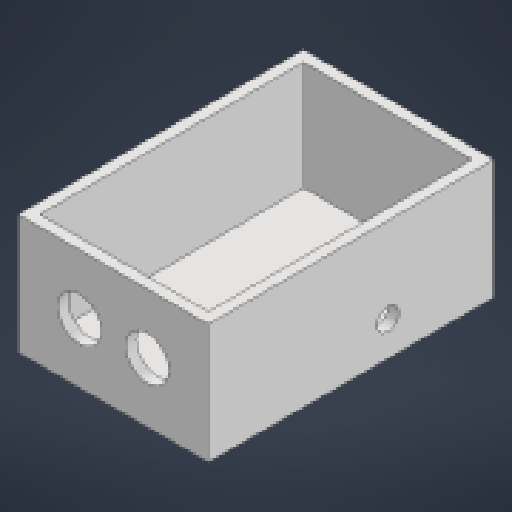
# Autodesk Inventor part: Prototipo
Saved by Autodesk Inventor 2026 (Build 300175050, 175E)
## iProperties
Created: 2025-09-06
Part Number: Prototipo
Material: Genérico
Document SubType Name: Modeling
Designer: alanl
Density: 1 g/cm^3
Appearance: Padrão
Author: alanl
Autodesk Inventor part; units mm, degrees
ref_plane "YZ Plane" through (0, 0, 0) normal (1, 0, 0) x (0, 1, 0)
ref_plane "XZ Plane" through (0, 0, 0) normal (0, 1, 0) x (-1, 0, 0)
ref_plane "XY Plane" through (0, 0, 0) normal (0, 0, 1) x (1, 0, 0)
sketch "Esboço1" plane through (0, 0, 0) normal (0, 1, 0) x (-1, 0, 0)
  line L0 (0, 0) -> (72, 0)
  line L1 (72, 0) -> (72, -110)
  line L2 (72, -110) -> (0, -110)
  line L3 (0, -110) -> (0, 0)
  dimension "d0" = 72
  dimension "d1" = 110
  constraints: 8 end point, 2 parallel, 1 horizontal, 1 perpendicular
  measures "d0" distance of L1.end L2.end
  measures "d1" distance of L0.end L1.end
extrude "Extrusão1" add sketch "Esboço1" along normal blind 6
sketch "Esboço2" plane through (0, 6, 0) normal (0, 1, 0) x (1, 0, 0)
  line L0 (0, 110) -> (-72, 110) projected
  line L1 (-72, 110) -> (-72, 0) projected
  line L2 (-72, 0) -> (0, 0) projected
  line L3 (0, 0) -> (0, 110) projected
  line L4 (-66, 104) -> (-6, 104)
  line L5 (-6, 104) -> (-6, 6)
  line L6 (-6, 6) -> (-66, 6)
  line L7 (-66, 6) -> (-66, 104)
  dimension "d4" = 6
  constraints: 8 end point, 3 other
  measures "d4" distance between parallel lines of L1 L7
extrude "Extrusão2" add sketch "Esboço2" along normal blind 44
sketch "Esboço3" plane through (-72, 0, 0) normal (0, 0, 1) x (1, 0, 0)
  circle A0 centre (23.5, 25) radius 8
  circle A1 centre (48.5, 25) radius 8
  line L0 (0, 50) -> (72, 50) projected
  line L1 (0, 0) -> (0, 50) projected
  line L2 (23.5, 25) -> (48.5, 25) construction
  point P0 (72, 0)
  point P1 (0, 25)
  point P2 (36, 25)
  point P3 (36, 50)
  dimension "d8" = 16
  dimension "d9" = 25
  constraints: 3 midpoint, 2 centre point, 2 end point, 2 horizontal alignment, 1 equal radius, 1 horizontal, 1 vertical alignment
  measures "d8" diameter of A0
  measures "d9" distance of L2.start L2.end
extrude "Extrusão3" cut sketch "Esboço3" against normal up to surface (6 mm away)
sketch "Esboço4" plane through (0, 0, 0) normal (1, 0, 0) x (0, 0, -1)
  line L0 (22.03, 11.6) -> (28.37, 11.6) projected
  arc A0 (28.37, 11.6) -> (29.67, 12.9) centre (28.37, 12.9) ccw projected
  line L1 (29.67, 12.9) -> (29.67, 13.46) projected
  arc A1 (29.67, 13.46) -> (28.37, 14.76) centre (28.37, 13.46) ccw projected
  line L2 (22.03, 14.76) -> (28.37, 14.76) projected
  arc A2 (22.03, 14.76) -> (20.73, 13.46) centre (22.03, 13.46) ccw projected
  line L3 (20.73, 12.9) -> (20.73, 13.46) projected
  arc A3 (20.73, 12.9) -> (22.03, 11.6) centre (22.03, 12.9) ccw projected
  arc A4 (28.37, 11.9) -> (29.37, 12.9) centre (28.37, 12.9) ccw projected
  line L4 (28.37, 11.9) -> (22.03, 11.9) projected
  arc A5 (21.03, 12.9) -> (22.03, 11.9) centre (22.03, 12.9) ccw projected
  line L5 (21.03, 13.46) -> (21.03, 12.9) projected
  arc A6 (22.03, 14.46) -> (21.03, 13.46) centre (22.03, 13.46) ccw projected
  line L6 (22.03, 14.46) -> (28.37, 14.46) projected
  arc A7 (29.37, 13.46) -> (28.37, 14.46) centre (28.37, 13.46) ccw projected
  line L7 (29.37, 12.9) -> (29.37, 13.46) projected
  line L8 (37.8445, 11.75) -> (39.84, 11.75) projected
  arc A8 (37.6268, 11.8436) -> (37.8445, 11.75) centre (37.8445, 12.05) ccw projected
  line L9 (36.9823, 12.5234) -> (37.6268, 11.8436) projected
  arc A9 (36.9, 12.7298) -> (36.9823, 12.5234) centre (37.2, 12.7298) ccw projected
  line L10 (36.9, 14.05) -> (36.9, 12.7298) projected
  arc A10 (37.2, 14.35) -> (36.9, 14.05) centre (37.2, 14.05) ccw projected
  line L11 (42.8, 14.35) -> (37.2, 14.35) projected
  arc A11 (43.1, 14.05) -> (42.8, 14.35) centre (42.8, 14.05) ccw projected
  line L12 (43.1, 12.7298) -> (43.1, 14.05) projected
  arc A12 (43.0177, 12.5234) -> (43.1, 12.7298) centre (42.8, 12.7298) ccw projected
  line L13 (42.3732, 11.8436) -> (43.0177, 12.5234) projected
  arc A13 (42.1555, 11.75) -> (42.3732, 11.8436) centre (42.1555, 12.05) ccw projected
  line L14 (40.16, 11.75) -> (42.1555, 11.75) projected
  line L15 (40.16, 11.6) -> (40.16, 11.75) projected
  line L16 (42.1555, 11.6) -> (40.16, 11.6) projected
  arc A14 (42.1555, 11.6) -> (42.4821, 11.7404) centre (42.1555, 12.05) ccw projected
  line L17 (43.1266, 12.4202) -> (42.4821, 11.7404) projected
  arc A15 (43.1266, 12.4202) -> (43.25, 12.7298) centre (42.8, 12.7298) ccw projected
  line L18 (43.25, 14.05) -> (43.25, 12.7298) projected
  arc A16 (43.25, 14.05) -> (42.8, 14.5) centre (42.8, 14.05) ccw projected
  line L19 (37.2, 14.5) -> (42.8, 14.5) projected
  arc A17 (37.2, 14.5) -> (36.75, 14.05) centre (37.2, 14.05) ccw projected
  line L20 (36.75, 12.7298) -> (36.75, 14.05) projected
  arc A18 (36.75, 12.7298) -> (36.8734, 12.4202) centre (37.2, 12.7298) ccw projected
  line L21 (37.5179, 11.7404) -> (36.8734, 12.4202) projected
  arc A19 (37.5179, 11.7404) -> (37.8445, 11.6) centre (37.8445, 12.05) ccw projected
  line L22 (39.84, 11.6) -> (37.8445, 11.6) projected
  line L23 (39.84, 11.75) -> (39.84, 11.6) projected
  line L24 (51.3445, 11.75) -> (53.34, 11.75) projected
  arc A20 (51.1268, 11.8436) -> (51.3445, 11.75) centre (51.3445, 12.05) ccw projected
  line L25 (50.4823, 12.5234) -> (51.1268, 11.8436) projected
  arc A21 (50.4, 12.7298) -> (50.4823, 12.5234) centre (50.7, 12.7298) ccw projected
  line L26 (50.4, 14.05) -> (50.4, 12.7298) projected
  arc A22 (50.7, 14.35) -> (50.4, 14.05) centre (50.7, 14.05) ccw projected
  line L27 (56.3, 14.35) -> (50.7, 14.35) projected
  arc A23 (56.6, 14.05) -> (56.3, 14.35) centre (56.3, 14.05) ccw projected
  line L28 (56.6, 12.7298) -> (56.6, 14.05) projected
  arc A24 (56.5177, 12.5234) -> (56.6, 12.7298) centre (56.3, 12.7298) ccw projected
  line L29 (55.8732, 11.8436) -> (56.5177, 12.5234) projected
  arc A25 (55.6555, 11.75) -> (55.8732, 11.8436) centre (55.6555, 12.05) ccw projected
  line L30 (53.66, 11.75) -> (55.6555, 11.75) projected
  line L31 (53.66, 11.6) -> (53.66, 11.75) projected
  line L32 (55.6555, 11.6) -> (53.66, 11.6) projected
  arc A26 (55.6555, 11.6) -> (55.9821, 11.7404) centre (55.6555, 12.05) ccw projected
  line L33 (56.6266, 12.4202) -> (55.9821, 11.7404) projected
  arc A27 (56.6266, 12.4202) -> (56.75, 12.7298) centre (56.3, 12.7298) ccw projected
  line L34 (56.75, 14.05) -> (56.75, 12.7298) projected
  arc A28 (56.75, 14.05) -> (56.3, 14.5) centre (56.3, 14.05) ccw projected
  line L35 (50.7, 14.5) -> (56.3, 14.5) projected
  arc A29 (50.7, 14.5) -> (50.25, 14.05) centre (50.7, 14.05) ccw projected
  line L36 (50.25, 12.7298) -> (50.25, 14.05) projected
  arc A30 (50.25, 12.7298) -> (50.3734, 12.4202) centre (50.7, 12.7298) ccw projected
  line L37 (51.0179, 11.7404) -> (50.3734, 12.4202) projected
  arc A31 (51.0179, 11.7404) -> (51.3445, 11.6) centre (51.3445, 12.05) ccw projected
  line L38 (53.34, 11.6) -> (51.3445, 11.6) projected
  line L39 (53.34, 11.75) -> (53.34, 11.6) projected
  line L40 (64.5, 17.6) -> (64.5, 11.6) projected
  line L41 (68, 11.6) -> (64.5, 11.6) projected
  arc A32 (68, 17.6) -> (68, 11.6) centre (68, 14.6) ccw projected
  line L42 (68, 17.6) -> (64.5, 17.6) projected
  line L43 (71.5, 17.6) -> (68, 17.6) projected
  arc A33 (68, 11.6) -> (68, 17.6) centre (68, 14.6) ccw projected
  line L44 (71.5, 11.6) -> (68, 11.6) projected
  line L45 (71.5, 11.6) -> (71.5, 17.6) projected
  circle A34 centre (68, 14.6) radius 4
  point P0 (0, 0)
  dimension "d12" = 1
  constraints: 1 centre point, 1 coincident
  measures "d12" radial gap between concentric circles of A33 A34
extrude "Extrusão4" cut sketch "Esboço4" against normal up to next contours A34 L42 A32 L41 L40 | L40 A34 | A34 L43 L42 | A33 A32 | L43 A34 L45 L44 A33 | L41 L44 A34 | A34 L45
sketch "Esboço6" plane through (0, 50, 0) normal (0, 1, 0) x (1, 0, 0)
  line L0 (-72, 110) -> (-72, 0) projected
  line L1 (-72, 0) -> (0, 0) projected
  line L2 (0, 0) -> (0, 110) projected
  line L3 (0, 110) -> (-72, 110) projected
  line L4 (-66, 104) -> (-6, 104) projected
  line L5 (-6, 104) -> (-6, 6) projected
  line L6 (-6, 6) -> (-66, 6) projected
  line L7 (-66, 6) -> (-66, 104) projected
extrude "Extrusão5" add sketch "Esboço6" against normal blind 6 contours L4 L5 L6 L7
sketch "Esboço7" plane through (0, 0, 0) normal (1, 0, 0) x (0, 0, -1)
  line L0 (0, 0) -> (110, 0) projected
  line L1 (6, 6) -> (104, 6) projected
  line L2 (35, 0) -> (75, 0)
  line L3 (75, 0) -> (75, 6)
  line L4 (75, 6) -> (35, 6)
  line L5 (35, 6) -> (35, 0)
  point P0 (55, 6)
  point P1 (35, 6)
  point P2 (75, 0)
  dimension "d17" = 40
  constraints: 8 end point, 2 midpoint, 2 parallel, 2 point on line, 1 horizontal, 1 perpendicular
  measures "d17" distance between parallel lines of L3 L5
extrude "Extrusão6" add sketch "Esboço7" along normal blind 35
fillet "Arredondamento1" radius 10 4 edges at (0, 3, -35) (0, 3, -75) (35, 3, -75) (35, 3, -35)
ref_plane "Plano de trabalho1" through (-36, 0, -110) normal (1, 0, 0) x (0, 0, -1)
sketch "Esboço8" plane through (0, 6, -25) normal (0, 1, 0) x (1, 0, 0)
  circle A0 centre (17.5, 30) radius 5
  arc A1 (25, 10) -> (35, 20) centre (25, 20) ccw projected
  line L0 (35, 40) -> (35, 20) projected
  arc A2 (35, 40) -> (25, 50) centre (25, 40) ccw projected
  line L1 (10, 50) -> (25, 50) projected
  arc A3 (0, 60) -> (10, 50) centre (10, 60) ccw projected
  line L2 (0, 0) -> (0, 60) projected
  arc A4 (10, 10) -> (0, 0) centre (10, 0) ccw projected
  line L3 (10, 10) -> (25, 10) projected
  point P0 (0, -25)
  point P1 (35, 30)
  point P2 (17.5, 50)
  dimension "d21" = 10
  constraints: 2 midpoint, 1 centre point, 1 horizontal alignment, 1 vertical alignment
  measures "d21" diameter of A0
extrude "Extrusão7" cut sketch "Esboço8" against normal blind 35 contours A0
mirror "Espelhar2" about plane through (-36, 0, -110) normal (1, 0, 0) of "Extrusão6", "Extrusão7"
fillet "Arredondamento2" radius 10 4 edges at (-72, 3, -35) (-107, 3, -35) (-107, 3, -75) (-72, 3, -75)
